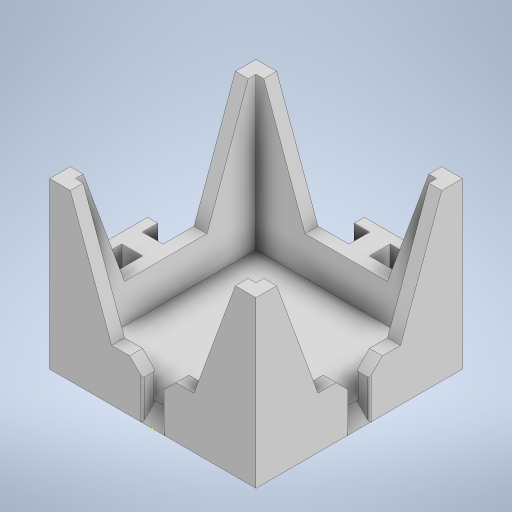
# Autodesk Inventor part: Checker square
Saved by Autodesk Inventor 2024 (Build 280153000, 153)
## iProperties
Created: 2024-03-17
Part Number: Checker square
Material: Generic
Document SubType Name: Modeling
Designer: drew
Density: 1 g/cm^3
Appearance: Default
Author: drew
Autodesk Inventor part; units mm, degrees
ref_plane "YZ Plane" through (0, 0, 0) normal (1, 0, 0) x (0, 1, 0)
ref_plane "XZ Plane" through (0, 0, 0) normal (0, 1, 0) x (-1, 0, 0)
ref_plane "XY Plane" through (0, 0, 0) normal (0, 0, 1) x (1, 0, 0)
sketch "Sketch1" plane through (0, 0, 0) normal (0, 1, 0) x (-1, 0, 0)
  point P0 (0, 0)
sketch "Sketch2" plane through (0, 0, 0) normal (0, 1, 0) x (-1, 0, 0)
  line L0 (-12.7, 12.7) -> (12.7, 12.7)
  line L1 (12.7, 12.7) -> (12.7, -12.7)
  line L2 (12.7, -12.7) -> (-12.7, -12.7)
  line L3 (-12.7, -12.7) -> (-12.7, 12.7)
  line L4 (-12.7, 12.7) -> (12.7, -12.7) construction
  line L5 (12.7, 12.7) -> (-12.7, -12.7) construction
  line L6 (3.175, -15.24) -> (-3.175, -15.24)
  line L7 (-3.175, -15.24) -> (-3.175, -16.51)
  line L8 (-3.175, -16.51) -> (3.175, -16.51)
  line L9 (3.175, -16.51) -> (3.175, -15.24)
  line L10 (3.175, -15.24) -> (-3.175, -16.51) construction
  line L11 (-3.175, -15.24) -> (3.175, -16.51) construction
  line L12 (-1.27, -15.24) -> (1.27, -15.24)
  line L13 (1.27, -15.24) -> (1.27, -12.7)
  line L14 (1.27, -12.7) -> (-1.27, -12.7)
  line L15 (-1.27, -12.7) -> (-1.27, -15.24)
  line L16 (15.24, 3.175) -> (15.24, -3.175)
  line L17 (15.24, -3.175) -> (16.51, -3.175)
  line L18 (16.51, -3.175) -> (16.51, 3.175)
  line L19 (16.51, 3.175) -> (15.24, 3.175)
  line L20 (15.24, 3.175) -> (16.51, -3.175) construction
  line L21 (15.24, -3.175) -> (16.51, 3.175) construction
  line L22 (15.24, 1.27) -> (12.7, 1.27)
  line L23 (12.7, -1.27) -> (15.24, -1.27)
  line L24 (12.7, 1.27) -> (12.7, -1.27)
  line L25 (3.175, 10.16) -> (-3.175, 10.16)
  line L26 (-3.175, 10.16) -> (-3.175, 8.89)
  line L27 (-3.175, 8.89) -> (3.175, 8.89)
  line L28 (3.175, 8.89) -> (3.175, 10.16)
  line L29 (3.175, 10.16) -> (-3.175, 8.89) construction
  line L30 (-3.175, 10.16) -> (3.175, 8.89) construction
  line L31 (-1.27, 10.16) -> (1.27, 10.16)
  line L32 (1.27, 10.16) -> (1.27, 12.7)
  line L33 (1.27, 12.7) -> (-1.27, 12.7)
  line L34 (-1.27, 12.7) -> (-1.27, 10.16)
  line L35 (-8.89, 3.175) -> (-10.16, 3.175)
  line L36 (-10.16, -1.27) -> (-10.16, 1.27)
  line L37 (-10.16, -3.175) -> (-8.89, 3.175) construction
  line L38 (-10.16, -3.175) -> (-8.89, -3.175)
  line L39 (-10.16, 3.175) -> (-10.16, -3.175)
  line L40 (-8.89, -3.175) -> (-8.89, 3.175)
  line L41 (-10.16, 3.175) -> (-8.89, -3.175) construction
  line L42 (-10.16, 1.27) -> (-12.7, 1.27)
  line L43 (-12.7, 1.27) -> (-12.7, -1.27)
  line L44 (-12.7, -1.27) -> (-10.16, -1.27)
  point P0 (0, 0)
  point P1 (0, -15.875)
  point P2 (15.875, 0)
  point P3 (0, 9.525)
  point P4 (-9.525, 0)
  point P5 (-1.27, 12.7)
  point P6 (-10.16, 1.27)
  point P7 (-12.7, -1.27)
  point P8 (-1.27, -12.7)
  point P9 (1.27, -15.24)
  dimension "d0" = 25.4
  dimension "d1" = 25.4
  dimension "d16" = 6.35
  dimension "d17" = 1.27
  dimension "d18" = 2.54
  dimension "d19" = 2.54
  dimension "d20" = 1.27
  dimension "d23" = 90
  dimension "d25" = 6.35
  dimension "d26" = 1.27
  dimension "d27" = 2.54
  dimension "d28" = 1.27
  dimension "d29" = 2.54
  dimension "d32" = 90
  constraints: 90 end point, 10 parallel, 6 midpoint, 5 horizontal, 5 perpendicular, 5 point on line, 2 vertical alignment, 1 collinear, 39 other
  measures "d0" distance of L1.end L2.end
  measures "d1" distance of L0.end L1.end
  measures "d16" distance of L8.end L7.end
  measures "d17" distance of L6.end L7.end
  measures "d18" distance between parallel lines of L2 L6
  measures "d19" distance between parallel lines of L15 L13
  measures "d20" distance from line of point (0, -15.875) L15
  measures "d25" distance of L28.start L27.start
  measures "d26" distance of L25.end L27.start
  measures "d27" distance between parallel lines of L34 L32
  measures "d28" distance from line of point (0, 9.525) L34
  measures "d29" distance between parallel lines of L0 L25
extrude "Extrusion1" add sketch "Sketch2" along normal blind 20.32 contours L0 L34 L25 L26 L27 L28 L32 L1 L2 L3 L44 L39 L38 L40 L35 L42 | L22 L16 L23 L1 | L2 L13 L6 L15 | L16 L19 L18 L17 | L6 L9 L8 L7
sketch "Sketch3" plane through (-12.7, 0, 12.7) normal (0, 0, 1) x (1, 0, 0)
  point P0 (12.7, 0)
sketch "Sketch4" plane through (-12.7, 0, 12.7) normal (0, 0, 1) x (1, 0, 0)
  line L0 (0, 20.32) -> (25.4, 20.32) projected
  line L1 (12.7, 0) -> (12.7, 20.32) construction
  line L2 (12.7, 6.35) -> (7.62, 6.35)
  line L3 (7.62, 6.35) -> (2.54, 20.32)
  line L4 (25.4, 20.32) -> (0, 20.32) projected
  line L5 (0, 0) -> (25.4, 0) projected
  line L6 (12.7, 6.35) -> (17.78, 6.35)
  line L7 (17.78, 6.35) -> (22.86, 20.32)
  dimension "d4" = 2.54
  dimension "d5" = 10.16
  dimension "d6" = 6.35
  constraints: 10 end point, 2 point on line, 2 symmetric about line, 1 horizontal, 1 midpoint
  measures "d4" distance of L0.start L3.end
  measures "d5" diameter of L2.end L1
  measures "d6" distance between parallel lines of L5 L2
extrude "Extrusion2" cut sketch "Sketch4" against normal through all
pattern_circular "Circular Pattern1" count 2 over 90 about axis through (0, -10, 0) along (0, 1, 0) of "Extrusion2"
sketch "Sketch5" plane through (-5.08, 6.35, 12.7) normal (0, 1, 0) x (1, 0, 0)
  point P0 (5.08, 12.7)
sketch "Sketch9" plane through (-12.7, 0, 12.7) normal (0, 0, 1) x (1, 0, 0)
  line L0 (11.43, 0) -> (0, 0) projected
  line L1 (0, 1) -> (-3.81, 4.81)
  line L2 (-3.81, 4.81) -> (-3.81, 0)
  line L3 (-3.81, 0) -> (-3.81, 6.35) projected
  line L4 (-3.81, 0) -> (0, 0)
  line L5 (0, 1) -> (0, 0)
  point P0 (12.7, 0)
  dimension "d34" = 0
  dimension "d35" = 45
  dimension "d50" = 1
  constraints: 8 end point, 2 perpendicular, 1 collinear
  measures "d34" distance between parallel lines of L3 L2
  measures "d35" angle of L4 L1
  measures "d50" distance of L1.start L0.end
extrude "Extrusion4" cut sketch "Sketch9" against normal through all
sketch "Sketch10" plane through (-12.7, 0, -12.7) normal (-1, 0, 0) x (0, 0, 1)
  line L0 (0, 0) -> (0, 6.35) projected
  line L1 (-3.81, 0) -> (-3.81, 6.35) projected
  line L2 (-3.81, 0) -> (0, 0)
  line L3 (-3.81, 4.81) -> (0, 1)
  line L4 (-3.81, 4.81) -> (-3.81, 3.81)
  point P0 (12.7, 0)
  dimension "d48" = 1
  dimension "d49" = 45
  constraints: 6 end point, 3 point on line, 1 collinear, 1 perpendicular
  measures "d48" distance from line of L2 L3.end
  measures "d49" angle of L2 L3
extrude "Extrusion5" cut sketch "Sketch10" against normal through all
sketch "Sketch11" plane through (1.27, 0, 12.7) normal (0, 0, 1) x (1, 0, 0)
  line L0 (11.43, 0) -> (11.43, 6.35) projected
  line L1 (0, 0) -> (11.43, 0) projected
  line L2 (11.43, 0) -> (7.62, 3.81)
  line L3 (7.62, 3.81) -> (7.62, 0)
  point P0 (-1.27, 0)
  dimension "d42" = 135
  constraints: 4 end point, 1 vertical
  measures "d42" angle of L1 L2
extrude "Extrusion6" add sketch "Sketch11" against normal up to surface (25.4 mm away)
sketch "Sketch12" plane through (12.7, 0, 12.7) normal (1, 0, 0) x (0, 0, -1)
  line L0 (0, 0) -> (2.54, 0) projected
  line L1 (0, 0) -> (3.81, 3.81)
  line L2 (3.81, 3.81) -> (3.81, 0)
  line L3 (0, 0) -> (0, 6.35) projected
  line L4 (0, 0) -> (3.81, 0)
  point P0 (12.7, 0)
  point P1 (3.81, 0)
  dimension "d45" = 45
  constraints: 6 end point, 1 coincident, 1 horizontal, 1 perpendicular
  measures "d45" angle of L0 L1
extrude "Extrusion7" add sketch "Sketch12" against normal up to surface (25.4 mm away)
sketch "Sketch6" plane through (0, 20.32, 0) normal (0, 1, 0) x (1, 0, 0)
  line L0 (11.1125, -11.1125) -> (-11.1125, -11.1125)
  line L1 (-11.1125, -11.1125) -> (-11.1125, 11.1125)
  line L2 (-11.1125, 11.1125) -> (11.1125, 11.1125)
  line L3 (11.1125, 11.1125) -> (11.1125, -11.1125)
  line L4 (11.1125, -11.1125) -> (-11.1125, 11.1125) construction
  line L5 (-11.1125, -11.1125) -> (11.1125, 11.1125) construction
  point P0 (0, 0)
  dimension "d12" = 22.225
  dimension "d13" = 22.225
  constraints: 12 end point, 2 midpoint, 2 parallel, 1 horizontal, 1 perpendicular
  measures "d12" distance of L1.end L2.end
  measures "d13" distance of L0.end L1.end
extrude "Extrusion3" cut sketch "Sketch6" against normal blind 18.7325
chamfer "Chamfer1" distance 1.5875 angle 45 4 edges at (1.27, 6.35, 11.9062) (-1.27, 6.35, 11.9062) (11.9062, 6.35, -1.27) (11.9062, 6.35, 1.27)
fillet "Fillet1" radius 0.2 8 edges at (12.7, 2.3812, 1.27) (11.1125, 3.175, 1.27) (1.27, 2.3812, 12.7) (1.27, 3.175, 11.1125) (-1.27, 2.3812, 12.7) (-1.27, 3.175, 11.1125) (11.1125, 3.175, -1.27) (12.7, 2.3812, -1.27)
body "Solid1"
